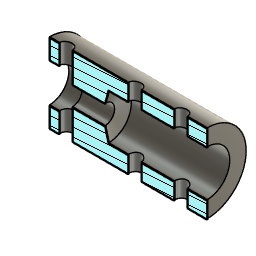
Pos19 (Autodesk Fusion 360 design; units mm, degrees)
Autodesk Fusion 360 part; units mm, degrees
sketch "Boceto1" plane through (0, 0, 0) normal (0, 1, 0) x (1, 0, 0)
  line L0 (0, -3) -> (0, -6)
  line L1 (0, -6) -> (24, -6)
  line L2 (24, -6) -> (24, -3.5)
  line L3 (24, -3.5) -> (9, -3.5)
  line L4 (9, -3.5) -> (8.4641, -1.5)
  line L5 (8.4641, -1.5) -> (3.5, -1.5)
  line L6 (3.5, -1.5) -> (3.5, -3)
  line L7 (0, -3) -> (3.5, -3)
  line L8 (0, 0) -> (32.7199, 0) construction
  dimension "d2" = 15
  dimension "d3" = 3.5
  dimension "d4" = 24
  dimension "d8" = 3
  dimension "d9" = 1.5
  dimension "d10" = 6
  dimension "d11" = 3.5
  dimension "d13" = 75
  constraint vertical L0
  constraint perpendicular L0 L1
  constraint perpendicular L1 L2
  constraint perpendicular L2 L3
  constraint perpendicular L2 L5
  constraint perpendicular L5 L6
  constraint perpendicular L6 L7
  constraint coincident L8.start origin
  constraint horizontal L8
  constraint vertical L8.start L0.start
  measures "d2" distance of L2.end L3.end
  measures "d3" distance of L0 L6.end
  measures "d4" distance of L0 L1.end
  measures "d8" vertical distance of L8.start L0.start
  measures "d9" vertical distance of L8.start L5.end
  measures "d10" vertical distance of L1.end L8.end
  measures "d11" distance of L2.end L8
  measures "d13" angle of L4 L5
  measures "d18" diameter of L5.end
revolve "Revolución1" add sketch "Boceto1" angle 360 about axis through (0, 0, 0) along (1, 0, 0)
sketch "Boceto2" plane through (0, 0, 0) normal (0, 0, 1) x (1, 0, 0)
  circle A0 centre (20, 0) radius 1
  circle A1 centre (13, 0) radius 1
  circle A2 centre (2.5, 0) radius 1
  point P0 (24, 0)
  dimension "d15" = 2.5
  dimension "d16" = 2
  dimension "d17" = 2
  dimension "d18" = 2
  dimension "d19" = 4
  dimension "d20" = 11
  measures "d15" distance of origin A2.centre
  measures "d16" diameter of A2
  measures "d17" diameter of A1
  measures "d18" diameter of A0
  measures "d19" distance of A0.centre P0
  measures "d20" distance of A1.centre P0
extrude "Extruir1" cut sketch "Boceto2" along normal mid plane 14
move_body "Move1" bodies 1 to x (1, 0, 0) y (0, 1, 0) z (0, 0, 1) at (0, 0, 6)
